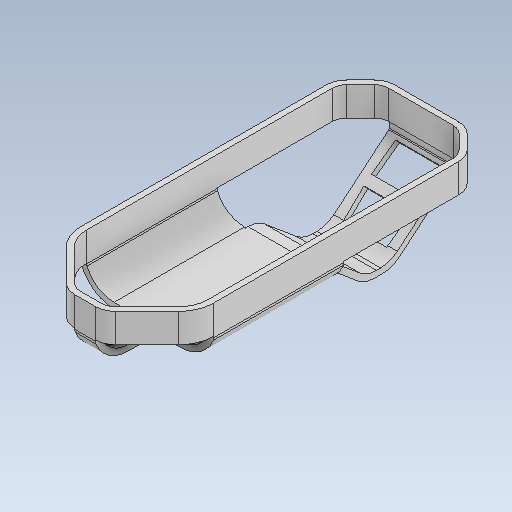
# Autodesk Inventor part: Enclosure Bottom
Saved by Autodesk Inventor 2020 (Build 240168000, 168)
## iProperties
Created: 2021-05-05
Part Number: Enclosure Bottom
Material: Generic
Document SubType Name: Modeling
Designer: Luke
Density: 1 g/cm^3
Appearance: Default
Author: Luke
Autodesk Inventor part; units mm, degrees
ref_plane "YZ Plane" through (0, 0, 0) normal (1, 0, 0) x (0, 1, 0)
ref_plane "XZ Plane" through (0, 0, 0) normal (0, 1, 0) x (-1, 0, 0)
ref_plane "XY Plane" through (0, 0, 0) normal (0, 0, 1) x (1, 0, 0)
sketch "Sketch1" plane through (0, 0, 0) normal (0, 1, 0) x (-1, 0, 0)
  line L0 (-21, -52.5168) -> (-21, 32.4844)
  line L1 (-18.0711, 39.5555) -> (-7.116, 50.5106)
  line L2 (-3.5804, 51.975) -> (3.6277, 51.975)
  line L3 (7.1632, 50.5106) -> (18.0082, 39.6656)
  line L4 (20.9372, 32.5945) -> (20.9371, -52.593)
  line L5 (19.4727, -56.1285) -> (14.6832, -60.918)
  line L6 (11.1477, -62.3824) -> (-11.1267, -62.3824)
  line L7 (-14.6594, -60.9208) -> (-19.5327, -56.0552)
  arc A0 (20.9372, 32.5945) -> (18.0082, 39.6656) centre (10.9372, 32.5945) ccw
  arc A1 (-18.0711, 39.5555) -> (-21, 32.4844) centre (-11, 32.4844) ccw
  arc A2 (-3.5804, 51.975) -> (-7.116, 50.5106) centre (-3.5804, 46.975) ccw
  arc A3 (7.1632, 50.5106) -> (3.6277, 51.975) centre (3.6277, 46.975) ccw
  arc A4 (19.4727, -56.1285) -> (20.9371, -52.593) centre (15.9371, -52.593) ccw
  arc A5 (11.1477, -62.3824) -> (14.6832, -60.918) centre (11.1477, -57.3824) ccw
  arc A6 (-14.6594, -60.9208) -> (-11.1267, -62.3824) centre (-11.1267, -57.3824) ccw
  arc A7 (-21, -52.5168) -> (-19.5327, -56.0552) centre (-16, -52.5168) ccw
  arc A8 (20.8869, -57.5427) -> (22.9371, -52.593) centre (15.9371, -52.593) ccw
  line L8 (22.9371, -52.593) -> (22.9371, 32.5945)
  arc A9 (22.9371, 32.5945) -> (19.4224, 41.0798) centre (10.9372, 32.5945) ccw
  line L9 (19.4224, 41.0798) -> (8.5774, 51.9248)
  arc A10 (8.5774, 51.9248) -> (3.6277, 53.975) centre (3.6277, 46.975) ccw
  line L10 (3.6277, 53.975) -> (-3.5804, 53.975)
  arc A11 (-3.5804, 53.975) -> (-8.5302, 51.9248) centre (-3.5804, 46.975) ccw
  line L11 (-8.5302, 51.9248) -> (-19.4853, 40.9697)
  arc A12 (-19.4853, 40.9697) -> (-23, 32.4844) centre (-11, 32.4844) ccw
  line L12 (-23, 32.4844) -> (-23, -52.5168)
  arc A13 (-23, -52.5168) -> (-20.9458, -57.4705) centre (-16, -52.5168) ccw
  line L13 (-20.9458, -57.4705) -> (-16.0725, -62.3361)
  arc A14 (-16.0725, -62.3361) -> (-11.1267, -64.3824) centre (-11.1267, -57.3824) ccw
  line L14 (-11.1267, -64.3824) -> (11.1477, -64.3824)
  arc A15 (11.1477, -64.3824) -> (16.0974, -62.3322) centre (11.1477, -57.3824) ccw
  line L15 (16.0974, -62.3322) -> (20.8869, -57.5427)
  line L16 (0.0236, 51.975) -> (112.4694, 51.975) construction
  line L17 (22.9371, -3.6687) -> (-23, -3.6687)
  line L18 (22.9371, -3.6687) -> (68.8743, -3.6687) construction
  point P0 (20.8869, -57.5427)
  dimension "d122" = 180
  constraints: 38 end point, 32 point on circle, 16 centre point, 2 horizontal, 2 point on line, 1 collinear, 1 midpoint, 15 other
  measures "d122" angle of L17 L18
extrude "Extrusion1" add sketch "Sketch1" along normal blind 10 contours A7 L7 A6 L6 A5 L5 A4 L4 L17 L8 A8 L15 A15 L14 A14 L13 A13 L12 L0 | L17 L12 A12 L11 A11 L10 A10 L9 A9 L8 L4 A0 L3 A3 L2 A2 L1 A1 L0
ref_plane "Work Plane7" through (-3.6277, 0, 0) normal (0, 0, 1) x (1, 0, 0)
ref_plane "Work Plane8" through (0.0314, 0, 32.4844) normal (1, 0, 0) x (0, 0, -1)
sketch "Sketch4" plane through (0.0314, 0, 32.4844) normal (1, 0, 0) x (0, 0, -1)
  line L0 (45.1952, -7) -> (45.9231, -7)
  line L1 (94.6882, -2.3125) -> (75.6597, -18.2793)
  line L2 (69.8746, -20.3849) -> (68.4261, -20.3849)
  line L3 (62.641, -18.2793) -> (51.7082, -9.1056)
  line L4 (50.9802, -11.1056) -> (61.913, -20.2793)
  line L5 (67.6981, -22.3849) -> (70.6025, -22.3849)
  line L6 (76.3876, -20.2793) -> (96.1524, -3.6947)
  line L7 (96.8668, 0) -> (96.8668, -2.1626)
  line L8 (94.8668, 0) -> (94.8668, -1.9295)
  arc A0 (50.9802, -11.1056) -> (45.1952, -9) centre (45.1952, -18) ccw
  arc A1 (51.7082, -9.1056) -> (45.9231, -7) centre (45.9231, -16) ccw
  arc A2 (69.8746, -20.3849) -> (75.6597, -18.2793) centre (69.8746, -11.3849) ccw
  arc A3 (62.641, -18.2793) -> (68.4261, -20.3849) centre (68.4261, -11.3849) ccw
  arc A4 (61.913, -20.2793) -> (67.6981, -22.3849) centre (67.6981, -13.3849) ccw
  arc A5 (70.6025, -22.3849) -> (76.3876, -20.2793) centre (70.6025, -13.3849) ccw
  arc A6 (96.1524, -3.6947) -> (96.8668, -2.1626) centre (94.8668, -2.1626) ccw
  line L9 (96.8668, 0) -> (94.8166, 0) projected
  line L10 (94.8668, 0) -> (96.8668, 0)
  arc A7 (94.6882, -2.3125) -> (94.8668, -1.9295) centre (94.3668, -1.9295) ccw
  line L11 (45.1952, -9) -> (45.1952, -7)
  line L12 (45.1952, -9) -> (47.1952, -9) construction
  point P0 (49.1988, -7)
  point P1 (94.8668, -2.1626)
  point P2 (73.1503, -20.3849)
  point P3 (65.1503, -20.3849)
  point P4 (48.4709, -9)
  point P5 (64.4224, -22.3849)
  point P6 (73.8783, -22.3849)
  point P7 (96.8668, -3.0952)
  dimension "d55" = 9
  dimension "d56" = 9
  dimension "d57" = 2
  dimension "d65" = 0.5
  dimension "d111" = 90
  constraints: 24 end point, 16 point on circle, 15 point on line, 15 tangent, 8 centre point, 4 equal radius, 3 horizontal, 1 perpendicular, 1 other
  measures "d55" radius of A0
  measures "d56" radius of A1
  measures "d57" radius of A6
  measures "d65" radius of A7
  measures "d111" angle of L12 L11
extrude "Extrusion3" add sketch "Sketch4" along normal mid plane 22
sketch "Sketch5" plane through (-10.9686, -3.0952, -64.3824) normal (0, -0.7660444, -0.6427876) x (1, 0, 0)
  line L0 (3.5641, 2.6135) -> (3.04, 12.6135) projected
  line L1 (18.5159, 2.6135) -> (3.5641, 2.6135) projected
  line L2 (19.04, 12.6135) -> (18.5159, 2.6135) projected
  line L3 (19.04, 12.6135) -> (3.04, 12.6135) projected
  line L4 (3.04, 16.3135) -> (19.04, 16.3135) projected
  line L5 (18.5159, 26.3135) -> (19.04, 16.3135) projected
  line L6 (3.5641, 26.3135) -> (18.5159, 26.3135) projected
  line L7 (3.04, 16.3135) -> (3.5641, 26.3135) projected
  line L8 (18.6583, 2.4635) -> (3.4217, 2.4635)
  line L9 (3.4217, 2.4635) -> (2.8819, 12.7635)
  line L10 (2.8819, 12.7635) -> (19.1981, 12.7635)
  line L11 (19.1981, 12.7635) -> (18.6583, 2.4635)
  line L12 (19.1981, 16.1635) -> (2.8819, 16.1635)
  line L13 (2.8819, 16.1635) -> (3.4217, 26.4635)
  line L14 (3.4217, 26.4635) -> (18.6583, 26.4635)
  line L15 (18.6583, 26.4635) -> (19.1981, 16.1635)
  point P0 (10.9686, 47.3302)
  dimension "d41" = 0.15
  dimension "d42" = 0.15
  constraints: 16 end point, 6 other
  measures "d41" distance between parallel lines of L2 L11
  measures "d42" distance between parallel lines of L4 L12
extrude "Extrusion4" cut sketch "Sketch5" against normal through all contours L0 L3 L2 L1 | L7 L6 L5 L4 | L8 L9 L10 L11 | L12 L13 L14 L15
ref_plane "Work Plane11" through (23, 0, -10.0162) normal (0, 0, -1) x (0, 1, 0)
ref_plane "Work Plane9" through (23, 0, 32.4844) normal (0, 0, -1) x (0, 1, 0)
ref_plane "Work Plane10" through (23, 0, -52.5168) normal (0, 0, -1) x (0, 1, 0)
sketch "Sketch6" plane through (23, 0, -10.0162) normal (0, 0, -1) x (0, 1, 0)
  line L0 (-7, -11.9686) -> (-7, -11.4686)
  line L1 (-7, -11.9686) -> (-6.5, -11.9686) construction
  line L2 (-9, -11.9686) -> (-9, -11.4686)
  line L3 (-9, -11.9686) -> (-8.5, -11.9686) construction
  line L4 (0, 0) -> (0.5, 0) construction
  line L5 (0, -2) -> (-0.2096, -2)
  line L6 (0, -2) -> (0.2096, -2) construction
  arc A0 (-0.7918, -2.1176) -> (-7, -11.4686) centre (3.1465, -11.4686) ccw
  arc A1 (-1.3265, -0.1757) -> (-9, -11.4686) centre (3.1465, -11.4686) ccw
  line L7 (-0.4058, 0) -> (0, 0)
  line L8 (0, 0) -> (0.5, 0)
  arc A2 (-0.2096, -2) -> (-0.7918, -2.1176) centre (-0.2096, -3.5) ccw
  arc A3 (-0.4058, 0) -> (-1.3265, -0.1757) centre (-0.4058, -2.5) ccw
  line L9 (0, -2.0542) -> (0, 0)
  line L10 (0, -2) -> (0, 0)
  line L11 (-9, -22.9686) -> (-7, -22.9686)
  line L12 (-7, -11.9686) -> (-7, -22.9686)
  line L13 (-9, -22.9686) -> (-9, -11.9686)
  point P0 (-0.5, -2)
  point P1 (-0.8546, 0)
  dimension "d89" = 0.5
  dimension "d90" = 90
  dimension "d91" = 0.5
  dimension "d92" = 90
  dimension "d95" = 0.5
  dimension "d96" = 180
  dimension "d97" = 2
  dimension "d98" = 1.5
  dimension "d99" = 2.5
  constraints: 28 end point, 10 point on circle, 4 centre point, 2 point on line
  measures "d89" distance of L0.start L0.end
  measures "d90" angle of L1 L0
  measures "d91" distance of L2.start L2.end
  measures "d92" angle of L3 L2
  measures "d95" distance of L5.start point (-0.5, -2)
  measures "d96" angle of L5 L6
  measures "d97" radial gap between concentric circles of A0 A1
  measures "d98" radius of A2
  measures "d99" radius of A3
extrude "Extrusion5" add sketch "Sketch6" along normal blind 2.695 and the other way blind 42.501
mirror "Mirror1" about plane through (0.0314, 0, 32.4844) normal (1, 0, 0) of "Extrusion5"
sketch "Sketch7" plane through (0.0314, 0, 32.4844) normal (1, 0, 0) x (0, 0, -1)
  line L0 (-9.5221, -7) -> (-10.0221, -7)
  line L1 (-9.5221, -9) -> (-10.0221, -9)
  line L2 (-19.4906, 0) -> (-19.4906, -0.2096)
  line L3 (-19.4906, 0) -> (-19.4906, 0.2096) construction
  arc A0 (-19.373, -0.7918) -> (-10.0221, -7) centre (-10.0221, 3.1465) ccw
  arc A1 (-21.315, -1.3265) -> (-10.0221, -9) centre (-10.0221, 3.1465) ccw
  line L4 (-21.4906, -0.4058) -> (-21.4906, 0)
  arc A2 (-19.4906, -0.2096) -> (-19.373, -0.7918) centre (-17.9906, -0.2096) ccw
  arc A3 (-21.4906, -0.4058) -> (-21.315, -1.3265) centre (-18.9906, -0.4058) ccw
  line L5 (-19.4365, 0) -> (-21.4906, 0)
  line L6 (-19.4906, 0) -> (-21.4906, 0)
  line L7 (1.4779, -9) -> (1.4779, -7)
  line L8 (-9.5221, -7) -> (1.4779, -7)
  line L9 (1.4779, -9) -> (-9.5221, -9)
  point P0 (32.4844, 0)
  point P1 (-19.4906, -0.5)
  point P2 (-21.4906, 0)
  dimension "d118" = 2
  constraints: 20 end point, 9 point on circle, 4 centre point, 1 point on line
  measures "d118" radial gap between concentric circles of A0 A1
extrude "Extrusion6" add sketch "Sketch7" along normal mid plane 7.208
body "Solid1"
